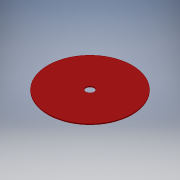
# Autodesk Inventor part: Sega Circolare 300 mm
Saved by Autodesk Inventor 2018 (Build 220112000, 112)
## iProperties
Created: 2020-06-01
Part Number: Sega Circolare 300 mm
Material: Acciaio
Document SubType Name: Modeling
Designer: Francesco
Density: 7.85 g/cm^3
Appearance: Rosso
Mass: 1139.36 g
Surface Area: 994 cm^2
Volume: 145.142 cm^3
Author: Francesco
Autodesk Inventor part; units mm, degrees
ref_plane "YZ Plane" through (0, 0, 0) normal (1, 0, 0) x (0, 1, 0)
ref_plane "XZ Plane" through (0, 0, 0) normal (0, 1, 0) x (-1, 0, 0)
ref_plane "XY Plane" through (0, 0, 0) normal (0, 0, 1) x (1, 0, 0)
sketch "Schizzo1" plane through (0, 0, 0) normal (0, 0, 1) x (1, 0, 0)
  circle A0 centre (0, 0) radius 150
  circle A1 centre (0, 0) radius 15
  dimension "d0" = 300
  dimension "d3" = 30
  constraints: 2 centre point, 2 coincident
  measures "d0" diameter of A0
  measures "d3" diameter of A1
extrude "Estrusione2" add sketch "Schizzo1" along normal blind 3
